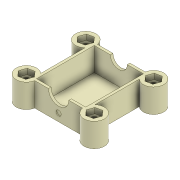
# Autodesk Inventor part: _UCHWYT_DUZY_SILNIK
Saved by Autodesk Inventor 2021 (Build 250183000, 183)
## iProperties
Created: 2022-11-28
Part Number: _UCHWYT_DUZY_SILNIK
Material: Generic
Document SubType Name: Modeling
Designer: agnpi
Density: 1 g/cm^3
Appearance: Smooth - Ash
Author: agnpi
Autodesk Inventor part; units mm, degrees
ref_plane "YZ Plane" through (0, 0, 0) normal (1, 0, 0) x (0, 1, 0)
ref_plane "XZ Plane" through (0, 0, 0) normal (0, 1, 0) x (-1, 0, 0)
ref_plane "XY Plane" through (0, 0, 0) normal (0, 0, 1) x (1, 0, 0)
sketch "Sketch1" plane through (0, 0, 0) normal (0, 1, 0) x (-1, 0, 0)
  line L0 (-14.5, 17) -> (14.5, 17)
  line L1 (14.5, 17) -> (14.5, -17)
  line L2 (14.5, -17) -> (-14.5, -17)
  line L3 (-14.5, -17) -> (-14.5, 17)
  line L4 (-14.5, 17) -> (14.5, -17) construction
  line L5 (14.5, 17) -> (-14.5, -17) construction
  circle A0 centre (-20, 17.5) radius 6
  circle A1 centre (20, 17.5) radius 6
  circle A2 centre (20, -17.5) radius 6
  circle A3 centre (-20, -17.5) radius 6
  line L6 (-16, 18.5) -> (16, 18.5)
  line L7 (16, 18.5) -> (16, -18.5)
  line L8 (16, -18.5) -> (-16, -18.5)
  line L9 (-16, -18.5) -> (-16, 18.5)
  line L10 (-16, 18.5) -> (16, -18.5) construction
  line L11 (16, 18.5) -> (-16, -18.5) construction
  point P0 (0, 0)
  point P1 (-16, -13.0279)
  point P2 (-14.0839, -18.5)
  point P3 (14.0839, -18.5)
  point P4 (16, -13.0279)
  point P5 (16, 13.0279)
  point P6 (14.0839, 18.5)
  point P7 (-14.0839, 18.5)
  point P8 (-16, 13.0279)
  point P9 (-14.5, -15.1021)
  point P10 (-14.0209, -17)
  point P11 (14.0209, -17)
  point P12 (14.5, -15.1021)
  point P13 (14.5, 15.1021)
  point P14 (14.0209, 17)
  point P15 (-14.0209, 17)
  point P16 (-14.5, 15.1021)
  dimension "d0" = 29
  dimension "d1" = 34
  dimension "d2" = 12
  dimension "d3" = 12
  dimension "d4" = 12
  dimension "d5" = 12
  dimension "d6" = 35
  dimension "d8" = 40
  dimension "d9" = 40
  dimension "d13" = 5.5
  dimension "d14" = 0.5
  dimension "d15" = 1.5
  dimension "d16" = 1.5
  constraints: 24 end point, 4 centre point, 4 midpoint, 4 parallel, 2 horizontal, 2 horizontal alignment, 2 perpendicular, 1 vertical alignment
  measures "d0" distance of L1.end L2.end
  measures "d1" distance of L0.end L1.end
  measures "d2" diameter of A0
  measures "d3" diameter of A1
  measures "d4" diameter of A2
  measures "d5" diameter of A3
  measures "d6" distance of A2.centre A1.centre
  measures "d8" distance of A2.centre A3.centre
  measures "d9" distance of A1.centre A0.centre
  measures "d13" distance from line of L1 A1.centre
  measures "d14" vertical distance of L0.end A1.centre
  measures "d15" distance between parallel lines of L0 L6
  measures "d16" distance between parallel lines of L7 L1
extrude "Extrusion1" add sketch "Sketch1" along normal blind 14 contours L3 A0 L9 L6 L0 | A0 L6 A1 L0 | L3 A3 L9 A0 | A1 L6 L7 L1 L0 | L3 L2 A3 L8 L9 | A0 L6 L9 | A1 L7 L6 | A1 L7 A2 L1 | L2 A2 L8 A3 | L9 L8 A3 | A2 L7 L8 L2 L1 | A2 L8 L7
extrude "Extrusion2" add sketch "Sketch1" along normal blind 0.2 contours L0 A1 L1 A2 L2 A3 L3 A0
hole "Hole1" at (-20, 0, -17.5) at (20, 0, -17.5) at (20, 0, 17.5) at (-20, 0, 17.5) direction (0, 1, 0) diameter 4 end through all
extrude "Extrusion3" add sketch "Sketch1" along normal blind 0.2 contours L0 A0 L3 | L0 L1 A1 | A3 L2 L3 | L1 L2 A2
sketch "Sketch2" plane through (0, 14, 0) normal (0, 1, 0) x (1, 0, 0)
  arc A0 (-16, -13.0279) -> (-14.0839, -18.5) centre (-20, -17.5) ccw projected
  line L0 (-17.3483, -20.5499) -> (-21.3155, -21.3214)
  line L1 (-21.3155, -21.3214) -> (-23.9671, -18.2714)
  line L2 (-23.9671, -18.2714) -> (-22.6517, -14.4501)
  line L3 (-22.6517, -14.4501) -> (-18.6845, -13.6786)
  line L4 (-18.6845, -13.6786) -> (-16.0329, -16.7286)
  line L5 (-16.0329, -16.7286) -> (-17.3483, -20.5499)
  line L6 (-10.7502, -12.1358) -> (-10.7502, 6.4156) construction
  line L7 (-10.7502, 6.4156) -> (-3.4446, 6.4156) construction
  line L8 (-22.6517, 20.5499) -> (-18.6845, 21.3214)
  line L9 (-18.6845, 21.3214) -> (-16.0329, 18.2714)
  line L10 (-16.0329, 18.2714) -> (-17.3483, 14.4501)
  line L11 (-17.3483, 14.4501) -> (-21.3155, 13.6786)
  line L12 (-21.3155, 13.6786) -> (-23.9671, 16.7286)
  line L13 (-23.9671, 16.7286) -> (-22.6517, 20.5499)
  line L14 (17.3483, -14.4501) -> (21.3155, -13.6786)
  line L15 (21.3155, -13.6786) -> (23.9671, -16.7286)
  line L16 (23.9671, -16.7286) -> (22.6517, -20.5499)
  line L17 (22.6517, -20.5499) -> (18.6845, -21.3214)
  line L18 (18.6845, -21.3214) -> (16.0329, -18.2714)
  line L19 (16.0329, -18.2714) -> (17.3483, -14.4501)
  line L20 (17.3483, 20.5499) -> (21.3155, 21.3214)
  line L21 (21.3155, 21.3214) -> (23.9671, 18.2714)
  line L22 (23.9671, 18.2714) -> (22.6517, 14.4501)
  line L23 (22.6517, 14.4501) -> (18.6845, 13.6786)
  line L24 (18.6845, 13.6786) -> (16.0329, 16.7286)
  line L25 (16.0329, 16.7286) -> (17.3483, 20.5499)
  point P0 (0, 0)
  dimension "d30" = 7
  dimension "d33" = 35
  dimension "d36" = 40
  constraints: 52 end point, 2 vertical, 1 coincident, 1 horizontal, 49 other
  measures "d30" distance between parallel lines of L0 L3
  measures "d33" distance of L2.end L8.start
  measures "d36" distance of L2.end L14.start
extrude "Extrusion4" cut sketch "Sketch2" against normal blind 3.2
sketch "Sketch3" plane through (-14.0839, 0, 18.5) normal (0, 0, 1) x (1, 0, 0)
  line L0 (28.1678, 14) -> (0, 14) projected
  arc A0 (8.0839, 14) -> (20.0839, 14) centre (14.0839, 14) ccw
  point P0 (14.0839, 0)
  dimension "d41" = 12
  constraints: 2 point on circle, 2 point on line, 1 centre point, 1 midpoint
  measures "d41" diameter of A0
extrude "Extrusion5" cut sketch "Sketch3" against normal up to surface (1.5 mm away)
sketch "Sketch4" plane through (-14.5, 14, -17) normal (0, 0, 1) x (1, 0, 0)
  line L0 (0, 0) -> (29, 0) projected
  arc A0 (9.5, 0) -> (19.5, 0) centre (14.5, 0) ccw
  point P0 (14.5, -14)
  dimension "d44" = 10
  constraints: 2 point on circle, 2 point on line, 1 centre point, 1 midpoint
  measures "d44" diameter of A0
extrude "Extrusion6" cut sketch "Sketch4" against normal through all
sketch "Sketch5" plane through (-14.0839, 0, 18.5) normal (0, 0, 1) x (1, 0, 0)
  circle A0 centre (14.0839, 4.5) radius 1.5
  line L0 (0, 0) -> (-11.9161, 0) projected
  point P0 (14.0839, 0)
  point P1 (-1.9161, 0)
  dimension "d47" = 3
  dimension "d48" = 4.5
  constraints: 1 centre point
  measures "d47" diameter of A0
  measures "d48" distance from line of L0 A0.centre
extrude "Extrusion7" cut sketch "Sketch5" against normal blind 0.5
body "Solid1"
